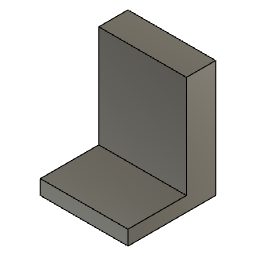
BTS7960 Housing Stands (Autodesk Fusion 360 design; units mm, degrees)
Autodesk Fusion 360 part; units mm, degrees
sketch "Sketch1" plane through (0, 0, 0) normal (0, 0, 1) x (1, 0, 0)
  line L0 (0, 0) -> (30, 0)
  line L1 (30, 0) -> (30, -30)
  line L2 (30, -30) -> (0, -30)
  line L3 (0, -30) -> (0, 0)
  dimension "d5" = 30
  dimension "d6" = 30
  constraint horizontal L0
  constraint vertical L1
  constraint horizontal L2
  constraint vertical L3
  constraint coincident L0.start L3.end
  measures "d5" distance of L0.start L2.end
  measures "d6" distance of L0.start L0.end
extrude "Extrude1" add sketch "Sketch1" along normal blind 5
sketch "Sketch2" plane through (0, 0, 5) normal (0, 0, 1) x (-1, 0, 0)
  line L0 (0, 30) -> (-30, 30)
  line L1 (-30, 30) -> (-30, 0)
  line L2 (-30, 0) -> (0, 0)
  line L3 (0, 0) -> (0, 30)
  line L4 (0, 0) -> (-30, 0)
  line L5 (-30, 0) -> (-30, 10)
  line L6 (-30, 10) -> (0, 10)
  line L7 (0, 10) -> (0, 0)
  dimension "d10" = 10
  dimension "d11" = 30
  constraint horizontal L4
  constraint vertical L5
  constraint horizontal L6
  constraint vertical L7
  constraint coincident L2.end L3.start
  measures "d10" distance of L2.end L6.end
  measures "d11" distance of L2.end L1.end
extrude "Extrude2" add sketch "Sketch2" along normal blind 35 contours L1 L2 L3 L4 L5 L6 L7
equation "base_sides = 30 mm"
equation "height = 40 mm"
equation "upper_length = 30 mm"
equation "upper_width = 10 mm"
equation "d5 = base_sides"
equation "d6 = base_sides"
equation "base_height = 5 mm"
equation "d8 = base_height"
equation "d10 = upper_width"
equation "d11 = upper_length"
equation "d12 = height - base_height"
